Autodesk Fusion 360 part; units mm, degrees
(part 9 of 9)
  spline S47 degree 5 poles (-7.5989, 1.7598) (-7.5979, 1.759) (-7.596, 1.7574) (-7.593, 1.755) (-7.5891, 1.7518) (-7.5843, 1.7478) (-7.5794, 1.7438) (-7.5746, 1.7398) (-7.5698, 1.7359) (-7.5649, 1.732) (-7.5601, 1.7281) (-7.5553, 1.7242) (-7.5505, 1.7204) (-7.5457, 1.7165) (-7.5409, 1.7127) (-7.5361, 1.7089) (-7.5313, 1.7052) (-7.5265, 1.7014) (-7.5218, 1.6977) (-7.517, 1.6939) (-7.5123, 1.6903) (-7.5075, 1.6866) (-7.5028, 1.6829) (-7.4981, 1.6793) (-7.4933, 1.6757) (-7.4886, 1.6721) (-7.4839, 1.6685) (-7.4792, 1.665) (-7.4746, 1.6614) (-7.4699, 1.6579) (-7.4652, 1.6544) (-7.4606, 1.6509) (-7.4559, 1.6475) (-7.4513, 1.6441) (-7.4466, 1.6406) (-7.442, 1.6373) (-7.4374, 1.6339) (-7.4328, 1.6305) (-7.4282, 1.6272) (-7.4236, 1.6239) (-7.419, 1.6206) (-7.4145, 1.6173) (-7.4099, 1.6141) (-7.4054, 1.6108) (-7.4008, 1.6076) (-7.3963, 1.6044) (-7.3918, 1.6012) (-7.3873, 1.5981) (-7.3828, 1.5949) (-7.3783, 1.5918) (-7.3738, 1.5887) (-7.3694, 1.5857) (-7.3649, 1.5826) (-7.3605, 1.5796) (-7.356, 1.5765) (-7.3516, 1.5735) (-7.3472, 1.5706) (-7.3428, 1.5676) (-7.3384, 1.5647) (-7.334, 1.5618) (-7.3297, 1.5589) (-7.3253, 1.556) (-7.321, 1.5531) (-7.3167, 1.5503) (-7.3123, 1.5475) (-7.308, 1.5447) (-7.3037, 1.5419) (-7.2994, 1.5391) (-7.2952, 1.5364) (-7.2909, 1.5336) (-7.2867, 1.5309) (-7.2824, 1.5283) (-7.2782, 1.5256) (-7.274, 1.5229) (-7.2698, 1.5203) (-7.2656, 1.5177) (-7.2615, 1.5151) (-7.2573, 1.5125) (-7.2532, 1.51) (-7.249, 1.5075) (-7.2449, 1.505) (-7.2408, 1.5025) (-7.2367, 1.5) (-7.2327, 1.4975) (-7.2286, 1.4951) (-7.2246, 1.4927) (-7.2205, 1.4903) (-7.2165, 1.4879) (-7.2125, 1.4855) (-7.2085, 1.4832) (-7.2045, 1.4809) (-7.2006, 1.4786) (-7.1966, 1.4763) (-7.1927, 1.474) (-7.1888, 1.4718) (-7.1849, 1.4696) (-7.181, 1.4674) (-7.1771, 1.4652) (-7.1733, 1.463) (-7.1694, 1.4608) (-7.1656, 1.4587) (-7.1618, 1.4566) (-7.158, 1.4545) (-7.1542, 1.4524) (-7.1504, 1.4504) (-7.1467, 1.4483) (-7.143, 1.4463) (-7.1393, 1.4443) (-7.1356, 1.4423) (-7.1319, 1.4403) (-7.1282, 1.4384) (-7.1246, 1.4365) (-7.1209, 1.4345) (-7.1173, 1.4326) (-7.1137, 1.4308) (-7.1101, 1.4289) (-7.1066, 1.4271) (-7.103, 1.4253) (-7.0995, 1.4234) (-7.096, 1.4217) (-7.0925, 1.4199) (-7.089, 1.4181) (-7.0856, 1.4164) (-7.0822, 1.4147) (-7.0787, 1.413) (-7.0753, 1.4113) (-7.072, 1.4097) (-7.0686, 1.408) (-7.0653, 1.4064) (-7.0619, 1.4048) (-7.0586, 1.4032) (-7.0553, 1.4016) (-7.0521, 1.4001) (-7.0488, 1.3985) (-7.0456, 1.397) (-7.0424, 1.3955) (-7.0392, 1.394) (-7.036, 1.3925) (-7.0329, 1.3911) (-7.0298, 1.3897) (-7.0267, 1.3882) (-7.0236, 1.3868) (-7.0205, 1.3855) (-7.0175, 1.3841) (-7.0144, 1.3827) (-7.0114, 1.3814) (-7.0085, 1.3801) (-7.0055, 1.3788) (-7.0026, 1.3775) (-6.9996, 1.3762) (-6.9967, 1.375) (-6.9939, 1.3738) (-6.991, 1.3726) (-6.9882, 1.3714) (-6.9854, 1.3702) (-6.9826, 1.369) (-6.9798, 1.3679) (-6.9771, 1.3667) (-6.9744, 1.3656) (-6.9717, 1.3645) (-6.969, 1.3634) (-6.9664, 1.3623) (-6.9638, 1.3613) (-6.9612, 1.3603) (-6.9586, 1.3592) (-6.956, 1.3582) (-6.9535, 1.3572) (-6.951, 1.3563) (-6.9485, 1.3553) (-6.9461, 1.3544) (-6.9436, 1.3534) (-6.9412, 1.3525) (-6.9388, 1.3516) (-6.9365, 1.3507) (-6.9342, 1.3499) (-6.9318, 1.349) (-6.9296, 1.3482) (-6.9273, 1.3474) (-6.9251, 1.3465) (-6.9229, 1.3458) (-6.9207, 1.345) (-6.9186, 1.3442) (-6.9164, 1.3435) (-6.9143, 1.3427) (-6.9123, 1.342) (-6.9102, 1.3413) (-6.9082, 1.3406) (-6.9062, 1.3399) (-6.9043, 1.3393) (-6.9023, 1.3386) (-6.9004, 1.338) (-6.8986, 1.3374) (-6.8967, 1.3368) (-6.8949, 1.3362) (-6.8931, 1.3356) (-6.8913, 1.335) (-6.8896, 1.3345) (-6.8879, 1.3339) (-6.8862, 1.3334) (-6.8846, 1.3329) (-6.883, 1.3324) (-6.8814, 1.3319) (-6.8798, 1.3314) (-6.8783, 1.331) (-6.8768, 1.3305) (-6.8753, 1.3301) (-6.8739, 1.3297) (-6.8725, 1.3293) (-6.8711, 1.3289) (-6.8698, 1.3285) (-6.8685, 1.3281) (-6.8672, 1.3278) (-6.866, 1.3274) (-6.8648, 1.3271) (-6.8636, 1.3268) (-6.8624, 1.3264) (-6.8613, 1.3261) (-6.8602, 1.3259) (-6.8592, 1.3256) (-6.8582, 1.3253) (-6.8572, 1.3251) (-6.8562, 1.3248) (-6.8553, 1.3246) (-6.8544, 1.3244) (-6.8536, 1.3241) (-6.8528, 1.3239) (-6.852, 1.3238) (-6.8513, 1.3236) (-6.8506, 1.3234) (-6.8499, 1.3232) (-6.8492, 1.3231) (-6.8487, 1.323) (-6.8481, 1.3228) (-6.8476, 1.3227) (-6.8471, 1.3226) (-6.8466, 1.3225) (-6.8462, 1.3224) (-6.8458, 1.3223) (-6.8455, 1.3223) (-6.8452, 1.3222) (-6.8449, 1.3221) (-6.8447, 1.3221) (-6.8446, 1.3221) (-6.8446, 1.3221) (-6.8445, 1.3221) knots -1 -1 -1 -1 -1 -1 -0.99583333 -0.99166667 -0.9875 -0.98333333 -0.97916667 -0.975 -0.97083333 -0.96666667 -0.9625 -0.95833333 -0.95416667 -0.95 -0.94583333 -0.94166667 -0.9375 -0.93333333 -0.92916667 -0.925 -0.92083333 -0.91666667 -0.9125 -0.90833333 -0.90416667 -0.9 -0.89583333 -0.89166667 -0.8875 -0.88333333 -0.87916667 -0.875 -0.87083333 -0.86666667 -0.8625 -0.85833333 -0.85416667 -0.85 -0.84583333 -0.84166667 -0.8375 -0.83333333 -0.82916667 -0.825 -0.82083333 -0.81666667 -0.8125 -0.80833333 -0.80416667 -0.8 -0.79583333 -0.79166667 -0.7875 -0.78333333 -0.77916667 -0.775 -0.77083333 -0.76666667 -0.7625 -0.75833333 -0.75416667 -0.75 -0.74583333 -0.74166667 -0.7375 -0.73333333 -0.72916667 -0.725 -0.72083333 -0.71666667 -0.7125 -0.70833333 -0.70416667 -0.7 -0.69583333 -0.69166667 -0.6875 -0.68333333 -0.67916667 -0.675 -0.67083333 -0.66666667 -0.6625 -0.65833333 -0.65416667 -0.65 -0.64583333 -0.64166667 -0.6375 -0.63333333 -0.62916667 -0.625 -0.62083333 -0.61666667 -0.6125 -0.60833333 -0.60416667 -0.6 -0.59583333 -0.59166667 -0.5875 -0.58333333 -0.57916667 -0.575 -0.57083333 -0.56666667 -0.5625 -0.55833333 -0.55416667 -0.55 -0.54583333 -0.54166667 -0.5375 -0.53333333 -0.52916667 -0.525 -0.52083333 -0.51666667 -0.5125 -0.50833333 -0.50416667 -0.5 -0.49583333 -0.49166667 -0.4875 -0.48333333 -0.47916667 -0.475 -0.47083333 -0.46666667 -0.4625 -0.45833333 -0.45416667 -0.45 -0.44583333 -0.44166667 -0.4375 -0.43333333 -0.42916667 -0.425 -0.42083333 -0.41666667 -0.4125 -0.40833333 -0.40416667 -0.4 -0.39583333 -0.39166667 -0.3875 -0.38333333 -0.37916667 -0.375 -0.37083333 -0.36666667 -0.3625 -0.35833333 -0.35416667 -0.35 -0.34583333 -0.34166667 -0.3375 -0.33333333 -0.32916667 -0.325 -0.32083333 -0.31666667 -0.3125 -0.30833333 -0.30416667 -0.3 -0.29583333 -0.29166667 -0.2875 -0.28333333 -0.27916667 -0.275 -0.27083333 -0.26666667 -0.2625 -0.25833333 -0.25416667 -0.25 -0.24583333 -0.24166667 -0.2375 -0.23333333 -0.22916667 -0.225 -0.22083333 -0.21666667 -0.2125 -0.20833333 -0.20416667 -0.2 -0.19583333 -0.19166667 -0.1875 -0.18333333 -0.17916667 -0.175 -0.17083333 -0.16666667 -0.1625 -0.15833333 -0.15416667 -0.15 -0.14583333 -0.14166667 -0.1375 -0.13333333 -0.12916667 -0.125 -0.12083333 -0.11666667 -0.1125 -0.10833333 -0.10416667 -0.1 -0.09583333 -0.09166667 -0.0875 -0.08333333 -0.07916667 -0.075 -0.07083333 -0.06666667 -0.0625 -0.05833333 -0.05416667 -0.05 -0.04583333 -0.04166667 -0.0375 -0.03333333 -0.02916667 -0.025 -0.02083333 -0.01666667 -0.0125 -0.00833333 -0.00416667 0 0 0 0 0 0
  line L94 (-6.8445, 1.3221) -> (-6.8442, 1.322)
  line L95 (-6.8442, 1.322) -> (-6.3329, 1.2232)
  circle A48 centre (0, 0) radius 2
  dimension "d7" = 4
  constraint coincident A0.centre A1.centre
  measures "d7" diameter of A48
extrude "Extrude3" cut sketch "Sketch4" against normal blind 3 contours A48 bodies 1
